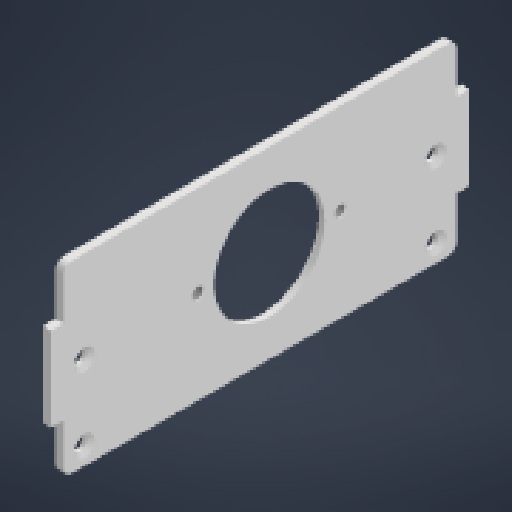
# Autodesk Inventor part: ściana
Saved by Autodesk Inventor 2026.1 (Build 301233020, 233B)
## iProperties
Created: 2026-02-27
Part Number: ściana
Material: Generic
Document SubType Name: Modeling
Designer: Jan
Density: 1 g/cm^3
Appearance: Default
Author: Jan
Autodesk Inventor part; units mm, degrees
ref_plane "YZ Plane" through (0, 0, 0) normal (1, 0, 0) x (0, 1, 0)
ref_plane "XZ Plane" through (0, 0, 0) normal (0, 1, 0) x (-1, 0, 0)
ref_plane "XY Plane" through (0, 0, 0) normal (0, 0, 1) x (1, 0, 0)
sketch "Sketch1" plane through (0, 0, 0) normal (1, 0, 0) x (0, 1, 0)
  line L0 (2, 0) -> (42, 0)
  line L1 (44, -2) -> (44, -92)
  line L2 (42, -94) -> (2, -94)
  line L3 (0, -92) -> (0, -2)
  line L4 (32, -94) -> (12, -94)
  line L5 (12, -94) -> (12, -97)
  line L6 (12, -97) -> (32, -97)
  line L7 (32, -97) -> (32, -94)
  line L8 (44.4582, -47) -> (27.4431, -47) construction
  line L9 (32, 0) -> (12, 0)
  line L10 (12, 0) -> (12, 3)
  line L11 (12, 3) -> (32, 3)
  line L12 (32, 3) -> (32, 0)
  arc A0 (42, -94) -> (44, -92) centre (42, -92) ccw
  arc A1 (0, -92) -> (2, -94) centre (2, -92) ccw
  arc A2 (2, 0) -> (0, -2) centre (2, -2) ccw
  arc A3 (44, -2) -> (42, 0) centre (42, -2) ccw
  point P0 (0, 0)
  point P1 (44, -94)
  point P2 (44, 0)
  point P3 (0, -94)
  point P4 (12, -95.5)
  point P5 (12, 1.5)
  dimension "d0" = 94
  dimension "d1" = 44
  dimension "d28" = 20
  dimension "d29" = 3
  dimension "d30" = 12
  dimension "d31" = 2
  constraints: 26 end point, 9 point on line, 8 point on circle, 8 tangent, 5 symmetric about line, 4 centre point, 4 parallel, 3 equal radius, 3 horizontal, 2 perpendicular, 1 midpoint
  measures "d0" distance of point (44, 0) point (44, -94)
  measures "d1" distance between parallel lines of L1 L3
  measures "d28" distance of L6.end L5.end
  measures "d29" distance of L5.end L4.end
  measures "d30" distance from line of point (12, -95.5) L3
  measures "d31" radius of A0
extrude "Extrusion1" add sketch "Sketch1" along normal blind 2
sketch "Sketch3" plane through (2, 0, 0) normal (1, 0, 0) x (0, 0, -1)
  circle A0 centre (49.25, 22) radius 13.2
  line L0 (0, 0) -> (92, 0) projected
  line L1 (94, 2) -> (94, 42) projected
  point P0 (120, 0)
  point P1 (120, 62)
  point P2 (94, 2)
  dimension "d23" = 26.4
  dimension "d24" = 22
  dimension "d25" = 44.75
  constraints: 1 centre point, 1 other
  measures "d23" diameter of A0
  measures "d24" distance from line of A0.centre L0
extrude "Extrusion2" cut sketch "Sketch3" against normal through all
sketch "Sketch4" plane through (2, 0, 0) normal (1, 0, 0) x (0, 0, -1)
  circle A0 centre (5, 22) radius 1.5
  circle A1 centre (89, 22) radius 1.5
  line L0 (2, 0) -> (92, 0) projected
  line L1 (92, 44) -> (2, 44) projected
  line L2 (0, 42) -> (0, 32) projected
  line L3 (94, 32) -> (94, 42) projected
  circle A2 centre (89, 4) radius 1.5
  circle A3 centre (5, 4) radius 1.5
  point P0 (0, 0)
  dimension "d32" = 3
  dimension "d33" = 3
  dimension "d34" = 44
  dimension "d35" = 22
  dimension "d36" = 5
  dimension "d37" = 5
  dimension "d62" = 3
  dimension "d63" = 3
  dimension "d64" = 18
  constraints: 4 centre point, 2 horizontal alignment, 2 vertical alignment
  measures "d32" diameter of A0
  measures "d33" diameter of A1
  measures "d34" distance between parallel lines of L0 L1
  measures "d35" distance from line of L1 A0.centre
  measures "d36" distance from line of A0.centre L2
  measures "d37" distance from line of L3 A1.centre
  measures "d62" diameter of A2
  measures "d63" diameter of A3
  measures "d64" distance of A2.centre A1.centre
hole "Hole2" at (2, 22, -5) at (2, 22, -89) at (2, 4, -89) at (2, 4, -5) direction (-1, 0, 0) diameter 3 depth 14.2 tip angle 118
chamfer "Chamfer2" distance 1 angle 45 4 edges at (2, 4, -87.5) (2, 22, -87.5) (2, 4, -3.5) (2, 22, -3.5)
sketch "Sketch5" plane through (2, 0, 0) normal (1, 0, 0) x (0, 0, -1)
  circle A0 centre (66.25, 22) radius 1.5
  circle A1 centre (32.25, 22) radius 1.5
  circle A2 centre (89, 22) radius 1.5 projected
  line L0 (89, 22) -> (83.0572, 22)
  circle A3 centre (49.25, 22) radius 13.2 projected
  point P0 (0, 0)
  point P1 (49.25, 8.8)
  dimension "d48" = 3
  dimension "d49" = 3
  dimension "d50" = 34
  dimension "d51" = 17
  constraints: 2 centre point, 2 end point, 2 horizontal alignment, 1 horizontal, 1 vertical alignment, 1 other
  measures "d48" diameter of A0
  measures "d49" diameter of A1
  measures "d50" distance of A1.centre A0.centre
  measures "d51" horizontal distance of point (49.25, 8.8) A0.centre
hole "Hole3" at (2, 22, -66.25) at (2, 22, -32.25) direction (-1, 0, 0) diameter 2.459 depth 8.8 tip angle 118 thread size "M3x0.5" class "6H" standard "ISO Metric profile"
chamfer "Chamfer3" distance 0.3 angle 45 2 edges at (2, 22, -65.0205) (2, 22, -31.0205)
chamfer "Chamfer4" distance 0.5 angle 45 1 edges at (0, 22, -36.05)
equation "\"d30\" = -0.5 * d28 + 0.5 * d1"
equation "\"d35\" = 0.5 * d34"
equation "\"d51\" = 0.5 * d50"
body "Solid1"
